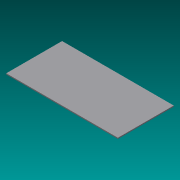
# Autodesk Inventor part: Patch Panel
Saved by Autodesk Inventor 2015 (Build 190159000, 159)
## iProperties
Created: 2015-06-05
Part Number: Patch Panel
Material: ABS Plastic
Document SubType Name: Modeling
Designer: Sawaiz Syed
Density: 1.06 g/cm^3
Appearance: Sky Blue Medium
Author: Sawaiz Syed
Autodesk Inventor part; units mm, degrees
ref_plane "YZ Plane" through (0, 0, 0) normal (1, 0, 0) x (0, 1, 0)
ref_plane "XZ Plane" through (0, 0, 0) normal (0, 1, 0) x (-1, 0, 0)
ref_plane "XY Plane" through (0, 0, 0) normal (0, 0, 1) x (1, 0, 0)
sketch "Sketch1" plane through (0, 0, 0) normal (0, 0, 1) x (1, 0, 0)
  line L0 (250, -125) -> (-250, -125)
  line L1 (-250, -125) -> (-250, 125)
  line L2 (-250, 125) -> (250, 125)
  line L3 (250, 125) -> (250, -125)
  line L4 (250, -125) -> (-250, 125) construction
  line L5 (-250, -125) -> (250, 125) construction
  point P0 (0, 0)
  dimension "d0" = 500
  dimension "d1" = 250
  constraints: 12 end point, 2 midpoint, 2 parallel, 1 horizontal, 1 perpendicular
  measures "d0" distance of L1.end L2.end
  measures "d1" distance of L0.end L1.end
extrude "Extrusion1" add sketch "Sketch1" along normal blind 4.7625
body "Solid1"
